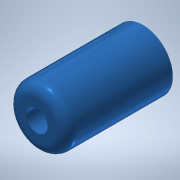
# Autodesk Inventor part: Fixador_Apoio_Rolamento
Saved by Autodesk Inventor 2022 (Build 260153000, 153)
## iProperties
Created: 2016-03-04
Part Number: Fixador_Apoio_Rolamento
Material: Genérico
Document SubType Name: Modeling
Designer: Everton
Density: 1 g/cm^3
Appearance: Padrão
Author: Everton
Autodesk Inventor part; units mm, degrees
ref_plane "YZ Plane" through (0, 0, 0) normal (1, 0, 0) x (0, 1, 0)
ref_plane "XZ Plane" through (0, 0, 0) normal (0, 1, 0) x (-1, 0, 0)
ref_plane "XY Plane" through (0, 0, 0) normal (0, 0, 1) x (1, 0, 0)
sketch "Sketch1" plane through (0, 0, 0) normal (0, 1, 0) x (-1, 0, 0)
  circle A0 centre (0, 0) radius 14
  dimension "d0" = 28
  constraints: 2 coincident, 1 centre point
  measures "d0" diameter of A0
extrude "Extrusion1" add sketch "Sketch1" along normal blind 50
sketch "Sketch2" plane through (0, 50, 0) normal (0, 1, 0) x (1, 0, 0)
  circle A0 centre (0, 0) radius 2.5
  dimension "d3" = 5
  constraints: 1 centre point, 1 coincident
  measures "d3" diameter of A0
hole "Hole1" at (0, 50, 0) direction (0, -1, 0) diameter 10.106 depth 50 tip angle 118 thread size "M12x1.75" class "6H" standard "ANSI Metric M Profile"
sketch "Sketch3" plane through (0, 0, 0) normal (1, 0, 0) x (0, 1, 0)
  line L0 (50, -14) -> (50, 14) projected
  line L1 (50, 14.1595) -> (0, -14)
  line L2 (0, 14) -> (0, -14) projected
  line L3 (50, 14.1595) -> (50, -14)
  line L4 (0, 14.1595) -> (15, 14.1595)
  line L5 (15, 14.1595) -> (15, 0.0798)
  circle A0 centre (15, 0.0798) radius 2
  point P0 (0, 0)
  dimension "d11" = 15
  dimension "d12" = 4
  constraints: 9 end point, 5 point on line, 2 perpendicular, 1 centre point, 1 coincident
  measures "d11" distance of L4.start L4.end
  measures "d12" diameter of A0
hole "Hole2" at (0, 15, 0.0798) direction (-1, 0, 0) diameter 6.647 depth 22.2 tip angle 118 thread size "M8x1.25" class "6H" standard "ANSI Metric M Profile"
fillet "Fillet1" radius 5 1 edges at (14, 0, 0)
body "Solid1"
